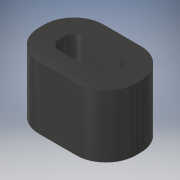
# Autodesk Inventor part: neues_bauteil
Saved by Autodesk Inventor 2017 (Build 210142000, 142)
## iProperties
Part Number: neues_bauteil
Material: Generisch
Document SubType Name: Modeling
Designer: Philomena-Theresa
Density: 1 g/cm^3
Appearance: Vorgabe
Author: Philomena-Theresa
Autodesk Inventor part; units mm, degrees
ref_plane "YZ Plane" through (0, 0, 0) normal (1, 0, 0) x (0, 1, 0)
ref_plane "XZ Plane" through (0, 0, 0) normal (0, 1, 0) x (-1, 0, 0)
ref_plane "XY Plane" through (0, 0, 0) normal (0, 0, 1) x (1, 0, 0)
sketch "Skizze1" plane through (0, 0, 0) normal (0, 0, 1) x (1, 0, 0)
  line L0 (-3.75, 6.5) -> (3.75, 6.5)
  line L1 (9.75, 0.5) -> (9.75, -0.5)
  line L2 (3.75, -6.5) -> (-3.75, -6.5)
  line L3 (-9.75, -0.5) -> (-9.75, 0.5)
  arc A0 (-3.75, 6.5) -> (-9.75, 0.5) centre (-3.75, 0.5) ccw
  arc A1 (-9.75, -0.5) -> (-3.75, -6.5) centre (-3.75, -0.5) ccw
  arc A2 (3.75, -6.5) -> (9.75, -0.5) centre (3.75, -0.5) ccw
  arc A3 (9.75, 0.5) -> (3.75, 6.5) centre (3.75, 0.5) ccw
  line L4 (3.75, 2.5) -> (-3.75, 2.5)
  arc A4 (-3.75, 2.5) -> (-5.75, 0.5) centre (-3.75, 0.5) ccw
  line L5 (-5.75, 0.5) -> (-5.75, -0.5)
  arc A5 (-5.75, -0.5) -> (-3.75, -2.5) centre (-3.75, -0.5) ccw
  line L6 (-3.75, -2.5) -> (3.75, -2.5)
  arc A6 (3.75, -2.5) -> (5.75, -0.5) centre (3.75, -0.5) ccw
  line L7 (5.75, -0.5) -> (5.75, 0.5)
  arc A7 (5.75, 0.5) -> (3.75, 2.5) centre (3.75, 0.5) ccw
  line L8 (-7.9926, 4.7426) -> (7.9926, -4.7426) construction
  point P0 (0, 0)
  point P1 (9.75, -6.5)
  point P2 (9.75, 6.5)
  point P3 (-9.75, -6.5)
  point P4 (0, 0)
  dimension "d0" = 19.5
  dimension "d1" = 13
  dimension "d2" = 6
  dimension "d3" = 6
  dimension "d4" = 6
  dimension "d5" = 4
  constraints: 18 end point, 18 point on circle, 8 centre point, 8 tangent, 6 point on line, 4 parallel, 2 perpendicular, 1 coincident, 1 equal radius, 1 horizontal, 1 midpoint, 7 other
  measures "d0" distance of point (9.75, -6.5) point (-9.75, -6.5)
  measures "d1" distance of point (9.75, 6.5) point (9.75, -6.5)
  measures "d2" radius of A0
  measures "d3" radius of A1
  measures "d4" radius of A3
  measures "d5" distance between parallel lines of L0 L4
extrude "Extrusion1" add sketch "Skizze1" along normal mid plane 12.6
